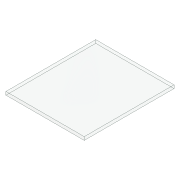
# Autodesk Inventor part: MiddleGlass
Saved by Autodesk Inventor 2020.3 (Build 243373010, 373A)
## iProperties
Created: 2020-12-04
Part Number: MiddleGlass
Material: Generic
Document SubType Name: Modeling
Designer: Yusuf
Mass: 42.218 g
Surface Area: 227.566 cm^2
Volume: 42.218 cm^3
Density: 1 g/cm^3
Appearance: Default
Author: Yusuf
Autodesk Inventor part; units mm, degrees
ref_plane "YZ Plane" through (0, 0, 0) normal (1, 0, 0) x (0, 1, 0)
ref_plane "XZ Plane" through (0, 0, 0) normal (0, 1, 0) x (-1, 0, 0)
ref_plane "XY Plane" through (0, 0, 0) normal (0, 0, 1) x (1, 0, 0)
sketch "Sketch1" plane through (0, 0, 0) normal (0, 1, 0) x (-1, 0, 0)
  line L0 (0, 0) -> (95.95, 0)
  line L1 (95.95, 0) -> (95.95, 110)
  line L2 (95.95, 110) -> (0, 110)
  line L3 (0, 110) -> (0, 0)
  dimension "d0" = 95.95
  dimension "d1" = 110
  constraints: 8 end point, 2 parallel, 1 horizontal, 1 perpendicular
  measures "d0" distance of L2.end L1.end
  measures "d1" distance of L0.end L1.end
extrude "Extrusion1" add sketch "Sketch1" along normal blind 4
body "Solid1"
